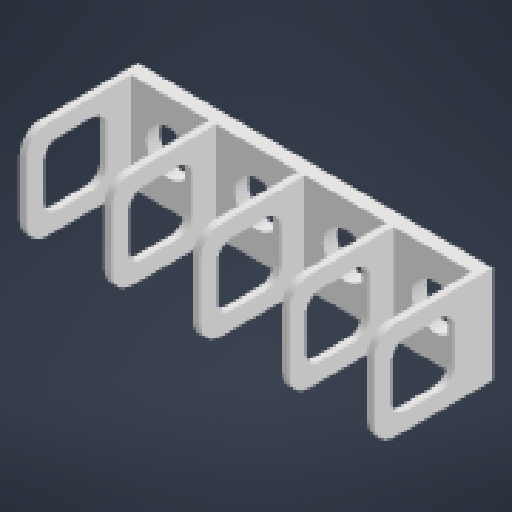
# Autodesk Inventor part: protector_small1x1
Saved by Autodesk Inventor 2024 (Build 280153000, 153)
## iProperties
Created: 2026-04-07
Part Number: protector_small1x1
Material: Generic
Document SubType Name: Modeling
Designer: schar
Density: 1 g/cm^3
Appearance: Light Red
Author: schar
Autodesk Inventor part; units mm, degrees
ref_plane "YZ Plane" through (0, 0, 0) normal (1, 0, 0) x (0, 1, 0)
ref_plane "XZ Plane" through (0, 0, 0) normal (0, 1, 0) x (-1, 0, 0)
ref_plane "XY Plane" through (0, 0, 0) normal (0, 0, 1) x (1, 0, 0)
sketch "Sketch1" plane through (0, 0, 0) normal (0, 0, 1) x (1, 0, 0)
  circle A0 centre (-19.0795, 0) radius 3.175 projected
  circle A1 centre (-6.3598, 0) radius 3.175 projected
  circle A2 centre (6.3597, 0) radius 3.175 projected
  circle A3 centre (19.0795, 0) radius 3.175 projected
  line L0 (25, -19) -> (25, 19) projected
  line L1 (-25, 19) -> (-25, -19) projected
  line L2 (-19.0795, 0) -> (-6.3598, 0)
  line L3 (-6.3598, 0) -> (-12.7197, 0)
  line L4 (-19.0795, 0) -> (-25.4395, 0)
  line L5 (19.0795, 0) -> (25.4395, 0)
  line L6 (-12.2197, 7) -> (-12.2197, -7)
  line L7 (-12.2197, -7) -> (-13.2197, -7)
  line L8 (-13.2197, -7) -> (-13.2197, 7)
  line L9 (-13.2197, 7) -> (-12.2197, 7)
  line L10 (-12.2197, 7) -> (-13.2197, -7) construction
  line L11 (-12.2197, -7) -> (-13.2197, 7) construction
  line L12 (-25.4395, 0) -> (-25.9395, 0)
  line L13 (-25.9395, 0) -> (-25.9395, 7)
  line L14 (25.4395, 0) -> (25.9395, 0)
  line L15 (25.9395, 0) -> (25.9395, -7)
  line L16 (-25.9395, 7) -> (25.9395, 7)
  line L17 (25.9395, 7) -> (25.9395, -7)
  line L18 (25.9395, -7) -> (-25.9395, -7)
  line L19 (-25.9395, -7) -> (-25.9395, 7)
  point P0 (0, 0)
  point P1 (-25, 7)
  point P2 (-25, -7)
  point P3 (25, -7)
  point P4 (25, 7)
  dimension "d0" = 6.36
  dimension "d1" = 6.36
  dimension "d2" = 14
  dimension "d3" = 1
  dimension "d4" = 0.5
  dimension "d5" = 7
  dimension "d6" = 0.5
  dimension "d7" = 7
  constraints: 36 end point, 5 horizontal, 5 perpendicular, 4 parallel, 3 midpoint, 1 point on line
  measures "d0" distance of L2.start L4.end
  measures "d1" distance of L5.start L5.end
  measures "d2" distance of L6.start L6.end
  measures "d3" distance of L6.end L7.end
  measures "d4" distance of L4.end L12.end
  measures "d5" distance of L12.end L13.end
  measures "d6" distance of L5.end L14.end
  measures "d7" distance of L14.end L15.end
extrude "Extrusion1" add sketch "Sketch1" along normal blind 2 contours L2 L8 L18 L1 L4 A0 | A0 L4 L1 L16 L8 L2 | L8 L9 L6 L2 | L2 L6 L7 L8 | L6 L16 L0 L18
sketch "Sketch2" plane through (0, 0, 2) normal (0, 0, 1) x (1, 0, 0)
  line L0 (-25, 7) -> (-24, 7)
  line L1 (25, 7) -> (-25, 7) projected
  circle A0 centre (-19.0795, 0) radius 3.175 projected
  circle A1 centre (-6.3598, 0) radius 3.175 projected
  line L2 (-19.0795, 0) -> (-6.3598, 0)
  line L3 (-13.2197, 7) -> (-13.2197, -7)
  line L4 (-13.2197, -7) -> (-12.2197, -7)
  line L5 (-12.2197, -7) -> (-12.2197, 7)
  line L6 (-12.2197, 7) -> (-13.2197, 7)
  line L7 (-13.2197, 7) -> (-12.2197, -7) construction
  line L8 (-13.2197, -7) -> (-12.2197, 7) construction
  line L9 (-0.5, 7) -> (-0.5, -7)
  line L10 (-0.5, -7) -> (0.5, -7)
  line L11 (0.5, -7) -> (0.5, 7)
  line L12 (0.5, 7) -> (-0.5, 7)
  line L13 (-0.5, 7) -> (0.5, -7) construction
  line L14 (-0.5, -7) -> (0.5, 7) construction
  circle A2 centre (6.3597, 0) radius 3.175 projected
  circle A3 centre (19.0795, 0) radius 3.175 projected
  line L15 (6.3597, 0) -> (19.0795, 0)
  line L16 (12.2196, 7) -> (12.2196, -7)
  line L17 (12.2196, -7) -> (13.2196, -7)
  line L18 (13.2196, -7) -> (13.2196, 7)
  line L19 (13.2196, 7) -> (12.2196, 7)
  line L20 (12.2196, 7) -> (13.2196, -7) construction
  line L21 (12.2196, -7) -> (13.2196, 7) construction
  line L22 (-24, 7) -> (-25, 7)
  line L23 (-25, 7) -> (-25, -7)
  line L24 (-25, -7) -> (-24, -7)
  line L25 (25, -7) -> (25, 7) projected
  line L26 (-25, -7) -> (25, -7) projected
  line L27 (25, 7) -> (24, 7)
  line L28 (24, 7) -> (24, -7)
  line L29 (24, -7) -> (25, -7)
  line L30 (25, -7) -> (25, 7)
  line L31 (-12.7197, 0) -> (-24.4397, 0)
  line L32 (-24.4397, 0) -> (-24.4397, 7)
  line L33 (-24.4397, 7) -> (-25.4397, 7)
  line L34 (-25.4397, 7) -> (-25.4397, -7)
  line L35 (-25.4397, -7) -> (-24.4397, -7)
  line L36 (-24.4397, -7) -> (-24.4397, 7)
  line L37 (0, 7) -> (0, -7)
  line L38 (25.4397, 7) -> (25.4397, -7)
  line L39 (25.4397, 7) -> (24.4397, 7)
  line L40 (24.4397, 7) -> (24.4397, -7)
  line L41 (24.4397, -7) -> (25.4397, -7)
  line L42 (25.4397, -7) -> (25.4397, 7)
  point P0 (0, 0)
  point P1 (12.7196, 0)
  dimension "d10" = 1
  dimension "d11" = 1
  dimension "d12" = 1
  dimension "d13" = 1
  dimension "d14" = 1
  dimension "d27" = 11.72
  dimension "d28" = 1
  dimension "d29" = 1
  constraints: 80 end point, 13 parallel, 10 perpendicular, 9 midpoint, 7 horizontal, 3 point on line, 2 symmetric about line, 3 other
  measures "d10" distance of L0.start L0.end
  measures "d11" distance of L4.end L3.end
  measures "d12" distance of L10.end L9.end
  measures "d13" distance of L17.end L16.end
  measures "d14" distance of L29.end L28.end
  measures "d27" distance of L31.start L31.end
  measures "d28" distance of L35.end L34.end
  measures "d29" distance of L41.end L40.end
extrude "Extrusion2" add sketch "Sketch2" along normal blind 15 contours L0 L32 L36 L24 L23 | L23 L35 L34 L33 | L1 L5 L2 L3 | L2 L5 L4 L3 | L1 L37 L10 L9 | L1 L11 L10 L37 | L1 L18 L15 L16 | L15 L18 L17 L16 | L1 L25 L26 L40 | L39 L38 L41 L25
sketch "Sketch3" plane through (-25, -7, 0) normal (-1, 0, 0) x (0, 0, 1)
  line L0 (2, 14) -> (2, 0) projected
  line L1 (0, 14) -> (2, 14) projected
  line L2 (0, 0) -> (2, 0) projected
  line L3 (14, 14) -> (3, 14)
  line L4 (3, 14) -> (3, 0)
  line L5 (3, 0) -> (14, 0)
  line L6 (17, 3) -> (17, 11)
  line L7 (7.5, 11.5) -> (12.5, 11.5)
  line L8 (14.5, 9.5) -> (14.5, 4.5)
  line L9 (12.5, 2.5) -> (7.5, 2.5)
  line L10 (5.5, 4.5) -> (5.5, 9.5)
  line L11 (5.5, 11.5) -> (14.5, 2.5) construction
  line L12 (14.5, 11.5) -> (5.5, 2.5) construction
  arc A0 (17, 11) -> (14, 14) centre (14, 11) ccw
  arc A1 (14, 0) -> (17, 3) centre (14, 3) ccw
  arc A2 (14.5, 9.5) -> (12.5, 11.5) centre (12.5, 9.5) ccw
  arc A3 (12.5, 2.5) -> (14.5, 4.5) centre (12.5, 4.5) ccw
  arc A4 (7.5, 11.5) -> (5.5, 9.5) centre (7.5, 9.5) ccw
  arc A5 (5.5, 4.5) -> (7.5, 2.5) centre (7.5, 4.5) ccw
  line L13 (17, 14) -> (17, 0) projected
  line L14 (0, 14) -> (2, 14) projected
  point P0 (0, 7)
  point P1 (10, 7)
  dimension "d18" = 14
  dimension "d19" = 9
  dimension "d20" = 9
  dimension "d21" = 3
  dimension "d22" = 3
  dimension "d23" = 2
  constraints: 20 end point, 13 point on line, 12 point on circle, 12 tangent, 6 centre point, 4 parallel, 3 equal radius, 2 horizontal, 2 midpoint, 2 perpendicular
  measures "d18" distance of point (17, 0) L4.end
  measures "d19" distance of L11.end L12.end
  measures "d20" distance of L12.start L11.end
  measures "d21" radius of A0
  measures "d22" radius of A1
  measures "d23" radius of A2
extrude "Extrusion3" cut sketch "Sketch3" against normal through all contours L7 A2 L8 A3 L9 A5 L10 A4
sketch "Sketch4" plane through (-25.4397, -7, 2) normal (-1, 0, 0) x (0, 0, 1)
  line L0 (0, 14) -> (0, 0)
  line L1 (-2, 14) -> (0, 14)
  line L2 (-2, 0) -> (0, 0)
  line L3 (12, 14) -> (1, 14)
  line L4 (1, 14) -> (1, 0)
  line L5 (1, 0) -> (12, 0)
  line L6 (15, 3) -> (15, 11)
  line L7 (5.5, 11.5) -> (10.5, 11.5)
  line L8 (12.5, 9.5) -> (12.5, 4.5)
  line L9 (10.5, 2.5) -> (5.5, 2.5)
  line L10 (3.5, 4.5) -> (3.5, 9.5)
  line L11 (3.5, 11.5) -> (12.5, 2.5) construction
  line L12 (12.5, 11.5) -> (3.5, 2.5) construction
  arc A0 (15, 11) -> (12, 14) centre (12, 11) ccw
  arc A1 (12, 0) -> (15, 3) centre (12, 3) ccw
  arc A2 (12.5, 9.5) -> (10.5, 11.5) centre (10.5, 9.5) ccw
  arc A3 (10.5, 2.5) -> (12.5, 4.5) centre (10.5, 4.5) ccw
  arc A4 (5.5, 11.5) -> (3.5, 9.5) centre (5.5, 9.5) ccw
  arc A5 (3.5, 4.5) -> (5.5, 2.5) centre (5.5, 4.5) ccw
  line L13 (15, 14) -> (15, 0)
  line L14 (-2, 14) -> (0, 14)
  line L15 (-2, 0) -> (0, 0) projected
  line L16 (-2, 0) -> (15, 0)
  line L17 (15, 0) -> (15, 14)
  line L18 (15, 14) -> (-2, 14)
  line L19 (-2, 14) -> (-2, 0)
  point P0 (-2, 7)
  point P1 (-2, 7)
  point P2 (15, 0)
  point P3 (8, 7)
  point P4 (12, 0)
  dimension "d30" = 14
  dimension "d31" = 9
  dimension "d32" = 9
  dimension "d33" = 3
  dimension "d34" = 3
  dimension "d35" = 2
  constraints: 38 end point, 13 point on line, 12 point on circle, 12 tangent, 6 centre point, 6 parallel, 3 equal radius, 3 horizontal, 3 perpendicular, 2 midpoint
  measures "d30" distance of point (15, 0) L5.start
  measures "d31" distance of L11.end L12.end
  measures "d32" distance of L12.start L11.end
  measures "d33" radius of A0
  measures "d34" radius of A1
  measures "d35" radius of A2
extrude "Extrusion4" cut sketch "Sketch4" against normal through all contours L18 L13 A0 | A1 L13 L16 | L7 A2 L8 A3 L9 A5 L10 A4
sketch "Sketch5" plane through (-25, -7, 0) normal (-1, 0, 0) x (0, 0, 1)
  line L0 (2, 14) -> (2, 0) projected
  line L1 (0, 14) -> (2, 14) projected
  line L2 (0, 0) -> (0, 14) projected
  line L3 (2, 14) -> (0, 14)
  line L4 (0, 14) -> (0, 0)
  line L5 (0, 0) -> (2, 0)
  line L6 (2, 0) -> (2, 14)
  point P0 (0, 7)
  point P1 (2, 0)
  constraints: 8 end point, 2 parallel, 1 horizontal, 1 perpendicular
extrude "Extrusion5" add sketch "Sketch5" along normal up to surface (0.4397 mm away)
sketch "Sketch6" plane through (25, -7, 0) normal (1, 0, 0) x (0, 0, -1)
  line L0 (-2, 0) -> (-2, 14) projected
  line L1 (0, 0) -> (0, 14) projected
  line L2 (0, 0) -> (0, 14) projected
  line L3 (0, 14) -> (-2, 14) projected
  line L4 (-2, 0) -> (-2, 14) projected
  line L5 (0, 0) -> (-2, 0) projected
  point P0 (0, 7)
extrude "Extrusion6" add sketch "Sketch6" along normal up to surface (0.4397 mm away)
body "Solid1"
